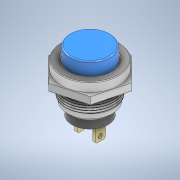
# Autodesk Inventor part: Кнопка2
Saved by Autodesk Inventor 2020 (Build 240168000, 168)
## iProperties
Created: 2020-02-08
Part Number: Кнопка2
Material: Типовые
Document SubType Name: Modeling
Designer: Andre
Density: 1 g/cm^3
Appearance: По умолчанию
Author: Andre
Autodesk Inventor part; units mm, degrees
ref_plane "YZ Plane" through (0, 0, 0) normal (1, 0, 0) x (0, 1, 0)
ref_plane "XZ Plane" through (0, 0, 0) normal (0, 1, 0) x (-1, 0, 0)
ref_plane "XY Plane" through (0, 0, 0) normal (0, 0, 1) x (1, 0, 0)
sketch "Эскиз1" plane through (0, 0, 0) normal (0, 1, 0) x (-1, 0, 0)
  circle A0 centre (0, 0) radius 6
  dimension "d0" = 12
  constraints: 1 centre point, 1 coincident
  measures "d0" diameter of A0
extrude "Выдавливание1" add sketch "Эскиз1" along normal mid plane 3
sketch "Эскиз2" plane through (0, -1.5, 0) normal (0, -1, 0) x (1, 0, 0)
  line L0 (-3.4, 1.7) -> (-2.6, 1.7)
  line L1 (-2.6, 1.7) -> (-2.6, -1.7)
  line L2 (-2.6, -1.7) -> (-3.4, -1.7)
  line L3 (-3.4, -1.7) -> (-3.4, 1.7)
  line L4 (-2.6, -1.7) -> (-3, -1.7)
  line L5 (2.6, 1.7) -> (3.4, 1.7)
  line L6 (3.4, 1.7) -> (3.4, -1.7)
  line L7 (3.4, -1.7) -> (2.6, -1.7)
  line L8 (2.6, -1.7) -> (2.6, 1.7)
  line L9 (3.4, -1.7) -> (3, -1.7)
  point P0 (0, 0)
  dimension "d5" = 0.8
  dimension "d6" = 3.4
  dimension "d9" = 0.8
  dimension "d10" = 3.4
  constraints: 20 end point, 4 parallel, 2 horizontal, 2 midpoint, 2 perpendicular
  measures "d5" distance of L1.end L2.end
  measures "d6" distance of L1.end L0.end
  measures "d9" distance of L6.end L7.end
  measures "d10" distance of L6.end L5.end
extrude "Выдавливание2" add sketch "Эскиз2" along normal blind 6
chamfer "Фаска1" distance 0.5 angle 45 4 edges at (-3, -7.5, -1.7) (3, -7.5, -1.7) (-3, -7.5, 1.7) (3, -7.5, 1.7)
sketch "Эскиз3" plane through (-3.4, -1.5, -1.7) normal (-1, 0, 0) x (0, 0, 1)
  line L0 (0.5, -6) -> (2.9, -6) projected
  line L1 (2.9, -6) -> (1.7, -6)
  line L2 (1.7, -6) -> (1.7, -4.5)
  circle A0 centre (1.7, -4.5) radius 0.75
  point P0 (1.7, 1.5)
  dimension "d20" = 1.2
  dimension "d21" = 1.5
  dimension "d22" = 1.5
  constraints: 4 end point, 1 centre point, 1 coincident, 1 midpoint, 1 perpendicular
  measures "d20" distance of L0.end L1.end
  measures "d21" distance of L1.end L2.end
  measures "d22" diameter of A0
hole "Отверстие1" at (-3.4, -6, 0) direction (1, 0, 0) diameter 1.5 end through all
sketch "Эскиз4" plane through (0, 1.5, 0) normal (0, 1, 0) x (1, 0, 0)
  circle A0 centre (0, 0) radius 7.5
  dimension "d31" = 15
  constraints: 1 centre point, 1 coincident
  measures "d31" diameter of A0
extrude "Выдавливание3" add sketch "Эскиз4" along normal blind 10
sketch "Эскиз19" plane through (0, 11.5, 0) normal (0, 1, 0) x (1, 0, 0)
  point P0 (0, 0)
sketch "Эскиз20" plane through (0, 11.5, 0) normal (0, 1, 0) x (1, 0, 0)
  circle A0 centre (0, 0) radius 8
  dimension "d111" = 16
  constraints: 1 centre point, 1 coincident
  measures "d111" diameter of A0
extrude "Выдавливание9" add sketch "Эскиз20" against normal blind 7.5
sketch "Эскиз21" plane through (0, 11.5, 0) normal (0, 1, 0) x (1, 0, 0)
  circle A0 centre (0, 0) radius 9.5
  dimension "d114" = 19
  constraints: 1 centre point, 1 coincident
  measures "d114" diameter of A0
extrude "Выдавливание10" add sketch "Эскиз21" along normal blind 1
thread "Резьба10" size "M16x0.75" class "6g" standard "ANSI Metric M Profile" full length
sketch "Эскиз23" plane through (0, 12.5, 0) normal (0, 1, 0) x (1, 0, 0)
  circle A0 centre (0, 0) radius 9.5
  circle A1 centre (0, 0) radius 9.5
  dimension "d120" = 19
  dimension "d121" = 19
  constraints: 2 centre point, 2 coincident
  measures "d120" diameter of A0
  measures "d121" diameter of A1
extrude "Выдавливание11" add sketch "Эскиз23" along normal blind 2
sketch "Эскиз25" plane through (0, 4, 0) normal (-1, 0, 0) x (0, 0, 1)
  line L0 (8, 0) -> (8, 7.5)
  line L1 (8, 7.5) -> (7.4439, 7.5)
  line L2 (7.4439, 7.5) -> (7.4439, 0)
  line L3 (7.4439, 0) -> (8, 0)
  line L4 (0, -15.9) -> (0, 14.9) projected
  constraints: 8 end point
revolve "Вращение5" cut sketch "Эскиз25" angle 360 about axis through (0, 4, 0) along (0, 1, 0)
sketch "Эскиз26" plane through (0, 4, 0) normal (-1, 0, 0) x (0, 0, 1)
  line L0 (8, 0) -> (8, 7.5)
  line L1 (8, 7.5) -> (7.4439, 7.5)
  line L2 (7.4439, 7.5) -> (7.4439, 0)
  line L3 (7.4439, 0) -> (8, 0)
  line L4 (0, -15.9) -> (0, 14.9) projected
  constraints: 8 end point
revolve "Вращение6" add sketch "Эскиз26" angle 360 about axis through (0, 4, 0) along (0, 1, 0) separate body
sketch "Эскиз24" plane through (0, 4, 0) normal (1, 0, 0) x (0, 1, 0)
  line L0 (-0.4376, -7.482) -> (-0.3751, -7.482) construction
  line L1 (0.0624, -7.9622) -> (-0.0001, -8.0823) construction
  line L2 (-0.7501, -8.0823) -> (-0.8126, -7.9622) construction
  line L3 (-0.3126, -7.482) -> (-0.3751, -7.3619) construction
  line L4 (-0.3751, -7.3619) -> (-0.4376, -7.482) construction
  line L5 (-0.7501, -8.0823) -> (-0.6876, -7.9622) construction
  line L6 (-0.3126, -7.482) -> (-0.0626, -7.9622)
  line L7 (-0.8126, -7.9622) -> (-0.6876, -7.9622) construction
  arc A0 (-0.8126, -7.9622) -> (-0.7501, -8.0002) centre (-0.7501, -7.9297) ccw construction
  line L8 (0.0624, -7.9622) -> (-0.0626, -7.9622) construction
  line L9 (-0.7501, -8.0823) -> (-0.7501, -7.9622) construction
  line L10 (-0.0001, -8.0823) -> (-0.0001, -7.9622) construction
  line L11 (-0.3751, -7.3619) -> (-0.3751, -7.4441) construction
  line L12 (-0.7501, -8.0002) -> (-0.0001, -8.0002)
  arc A1 (-0.7501, -8.0002) -> (-0.6876, -7.9622) centre (-0.7501, -7.9297) ccw
  line L13 (-0.0626, -7.9622) -> (-0.0001, -8.0823) construction
  line L14 (-0.6876, -7.9622) -> (-0.4376, -7.482)
  line L15 (-0.0001, -0.0002) -> (-0.0001, 0.0177)
  line L16 (-0.0001, 0.0177) -> (-0.0001, -0.0002)
  line L17 (-0.0001, -0.0002) -> (0.0334, -0.0002)
  arc A2 (-0.0626, -7.9622) -> (-0.0001, -8.0002) centre (-0.0001, -7.9297) ccw
  arc A3 (-0.0001, -8.0002) -> (0.0624, -7.9622) centre (-0.0001, -7.9297) ccw construction
  arc A4 (-0.3751, -7.4441) -> (-0.4376, -7.482) centre (-0.3751, -7.5145) ccw
  arc A5 (-0.3126, -7.482) -> (-0.3751, -7.4441) centre (-0.3751, -7.5145) ccw
  line L18 (-0.3751, -7.4441) -> (-0.3751, -7.482) construction
  line L19 (-0.3751, -7.482) -> (-0.3126, -7.482) construction
  dimension "d124" = 55
  dimension "d125" = 0.1201
  dimension "d126" = 0.1201
  dimension "Эскиз24_ThreadOffset" = 0
  dimension "Эскиз24_MajorRadius" = 8
  dimension "d129" = 0.75
  dimension "Эскиз24_MinorRadius" = 7.4439
  constraints: 40 end point, 12 point on circle, 10 parallel, 8 tangent, 6 centre point, 6 collinear, 2 midpoint, 2 point on line, 1 horizontal, 1 perpendicular, 3 other
  measures "d124" angle of L6 L14
  measures "d125" distance of L3.end L0.end
  measures "d126" distance of L1.end L10.end
  measures "Эскиз24_ThreadOffset" distance between parallel lines of L15 L10
  measures "Эскиз24_MajorRadius" distance from line of L12 L15.start
  measures "d129" distance from line of L1.end L9
  measures "Эскиз24_MinorRadius" distance edge to line of A5 L17
coil "Пружина3" sketch "Эскиз24" operation cut axis through (0, 4, 0) along (0, 1, 0) pitch 0.7508 turns 11.988012 hand right bodies 2
sketch "Эскиз27" plane through (0, 11.5, 0) normal (0, -1, 0) x (1, 0, 0)
  line L0 (-8.0081, -7.8676) -> (-10.8176, 3.0014)
  line L1 (-10.8176, 3.0014) -> (-2.8095, 10.8691)
  line L2 (-2.8095, 10.8691) -> (8.0081, 7.8676)
  line L3 (8.0081, 7.8676) -> (10.8176, -3.0014)
  line L4 (10.8176, -3.0014) -> (2.8095, -10.8691)
  line L5 (2.8095, -10.8691) -> (-8.0081, -7.8676)
  point P0 (0, 0)
  point P1 (0, 0)
  constraints: 12 end point, 1 coincident, 13 other
extrude "Выдавливание12" add sketch "Эскиз27" along normal blind 2.5 bodies 1
fillet "Сопряжение3" radius 0.2 6 edges at (-9.4129, 9, -2.4331) (-2.5993, 9, -9.3684) (-6.8136, 9, 6.9352) (2.5993, 9, 9.3684) (9.4129, 9, 2.4331) (6.8136, 9, -6.9352)
sketch "Эскиз28" plane through (0, 14.5, 0) normal (0, 1, 0) x (1, 0, 0)
  circle A0 centre (0, 0) radius 6.9
  dimension "d146" = 13.8
  constraints: 1 centre point, 1 coincident
  measures "d146" diameter of A0
extrude "Выдавливание13" cut sketch "Эскиз28" against normal blind 2 bodies 1
fillet "Сопряжение4" radius 0.4 1 edges at (-6.9, 14.5, 0)
sketch "Эскиз29" plane through (0, 12.5, 0) normal (0, 1, 0) x (1, 0, 0)
  circle A0 centre (0, 0) radius 6.75
  dimension "d150" = 13.5
  constraints: 1 centre point, 1 coincident
  measures "d150" diameter of A0
extrude "Выдавливание14" add sketch "Эскиз29" along normal blind 6 bodies 1
fillet "Сопряжение5" radius 0.4 1 edges at (-6.75, 18.5, 0)
chamfer "Фаска3" distance 1 angle 45 1 edges at (-7.5, 1.5, 0)
fillet "Сопряжение6" radius 0.2 1 edges at (-9.5, 14.5, 0)
equation "\"d124\" = d131"
equation "\"d125\" = 0.160083 * Эскиз24_Pitch"
equation "\"d126\" = 0.160083 * Эскиз24_Pitch"
equation "\"d129\" = Эскиз24_Pitch"
equation "\"d72\" = 55deg"
equation "\"Эскиз13_Pitch\" = 0.75"
equation "\"d95\" = 55deg"
equation "\"Эскиз16_Pitch\" = 0.75"
equation "\"d131\" = 55deg"
equation "\"Эскиз24_Pitch\" = 0.75"
